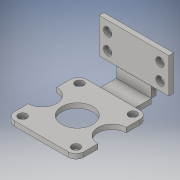
# Autodesk Inventor part: motor mount
Saved by Autodesk Inventor 2016 (Build 200138000, 138)
## iProperties
Created: 2017-09-13
Part Number: motor mount
Material: Generic
Document SubType Name: Modeling
Designer: student
Density: 1 g/cm^3
Appearance: Default
Author: student
Autodesk Inventor part; units mm, degrees
ref_plane "YZ Plane" through (0, 0, 0) normal (1, 0, 0) x (0, 1, 0)
ref_plane "XZ Plane" through (0, 0, 0) normal (0, 1, 0) x (-1, 0, 0)
ref_plane "XY Plane" through (0, 0, 0) normal (0, 0, 1) x (1, 0, 0)
sketch "Sketch1" plane through (0, 0, 0) normal (0, 0, 1) x (1, 0, 0)
  line L0 (-11.0744, 5.588) -> (11.0744, 5.588)
  line L1 (11.0744, 5.588) -> (11.0744, -5.588)
  line L2 (11.0744, -5.588) -> (-11.0744, -5.588)
  line L3 (-11.0744, -5.588) -> (-11.0744, 5.588)
  circle A0 centre (-8.3312, 2.4384) radius 1.3462
  circle A1 centre (8.3312, 2.4384) radius 1.3462
  circle A2 centre (8.3312, -2.794) radius 1.3462
  circle A3 centre (-8.3312, -2.794) radius 1.3462
  point P0 (0, 0)
  dimension "d0" = 22.1488
  dimension "d1" = 11.176
  dimension "d2" = 2.6924
  dimension "d3" = 2.6924
  dimension "d4" = 2.6924
  dimension "d5" = 2.6924
  dimension "d6" = 3.1496
  dimension "d7" = 2.794
  dimension "d8" = 5.2324
  dimension "d9" = 2.7432
  dimension "d10" = 2.7432
  dimension "d11" = 3.1496
  dimension "d12" = 2.794
  constraints: 8 end point, 4 centre point, 2 parallel, 2 vertical alignment, 1 horizontal, 1 perpendicular
  measures "d0" distance of L1.end L2.end
  measures "d1" distance of L1.end L0.end
  measures "d2" diameter of A0
  measures "d3" diameter of A1
  measures "d4" diameter of A2
  measures "d5" diameter of A3
  measures "d6" distance from line of L0 A1.centre
  measures "d7" distance from line of L2 A2.centre
  measures "d8" distance of A2.centre A1.centre
  measures "d9" distance from line of L1 A1.centre
  measures "d10" distance from line of L3 A0.centre
  measures "d11" vertical distance of L0.start A0.centre
  measures "d12" distance from line of L2 A3.centre
extrude "Extrusion1" add sketch "Sketch1" along normal blind 1.524
sketch "Sketch2" plane through (-11.0744, -5.588, 0) normal (0, -1, 0) x (1, 0, 0)
  line L0 (5.5245, 1.5517) -> (16.6243, 1.5517)
  line L1 (16.6243, 1.5517) -> (16.6243, 0.0277)
  line L2 (16.6243, 0.0277) -> (5.5245, 0.0277)
  line L3 (5.5245, 0.0277) -> (5.5245, 1.5517)
  point P0 (11.0744, 0)
  dimension "d15" = 11.0998
  dimension "d16" = 1.524
  constraints: 8 end point, 2 parallel, 1 horizontal, 1 perpendicular
  measures "d15" distance of L1.end L2.end
  measures "d16" distance of L1.end L0.end
extrude "Extrusion2" add sketch "Sketch2" along normal blind 3.3782
sketch "Sketch3" plane through (-5.5499, -5.588, 1.5517) normal (0, 0, 1) x (1, 0, 0)
  line L0 (0, -3.3922) -> (11.0998, -3.3922)
  line L1 (11.0998, -3.3922) -> (11.0998, -4.9162)
  line L2 (11.0998, -4.9162) -> (0, -4.9162)
  line L3 (0, -4.9162) -> (0, -3.3922)
  point P0 (5.5499, 5.588)
  dimension "d19" = 11.0998
  dimension "d20" = 1.524
  constraints: 8 end point, 2 parallel, 1 horizontal, 1 perpendicular
  measures "d19" distance of L1.end L2.end
  measures "d20" distance of L1.end L0.end
extrude "Extrusion3" add sketch "Sketch3" along normal blind 6.4008
sketch "Sketch4" plane through (-5.5499, -8.9802, 1.5517) normal (0, 1, 0) x (1, 0, 0)
  line L0 (14.0462, -29.432) -> (-2.9464, -29.432)
  line L1 (-2.9464, -6.5466) -> (14.0462, -6.5466)
  line L2 (-5.5245, 1.5517) -> (16.6243, 1.5517) projected
  arc A0 (-5.4864, -22.5228) -> (-5.4864, -13.4559) centre (-5.5498, -17.9893) ccw
  arc A1 (16.5862, -13.4558) -> (16.5862, -22.5229) centre (16.6412, -17.9893) ccw
  line L3 (16.5862, -9.0866) -> (16.5862, -13.4558)
  line L4 (16.5862, -22.5229) -> (16.5862, -26.892)
  line L5 (-5.4864, -26.892) -> (-5.4864, -22.5228)
  line L6 (-5.4864, -13.4559) -> (-5.4864, -9.0866)
  circle A2 centre (5.5499, -17.9893) radius 4.9657
  arc A3 (14.0462, -29.432) -> (16.5862, -26.892) centre (14.0462, -26.892) ccw
  arc A4 (-5.4864, -26.892) -> (-2.9464, -29.432) centre (-2.9464, -26.892) ccw
  arc A5 (16.5862, -9.0866) -> (14.0462, -6.5466) centre (14.0462, -9.0866) ccw
  arc A6 (-2.9464, -6.5466) -> (-5.4864, -9.0866) centre (-2.9464, -9.0866) ccw
  circle A7 centre (14.0462, -26.892) radius 1.3208
  circle A8 centre (14.0462, -8.8085) radius 1.3208
  circle A9 centre (-2.9464, -8.8085) radius 1.3208
  circle A10 centre (-2.9464, -26.892) radius 1.3208
  point P0 (5.5499, 1.5517)
  point P1 (-5.4864, -6.5466)
  point P2 (-5.4864, -29.432)
  point P3 (16.5862, -6.5466)
  point P4 (5.5499, 1.5517)
  point P5 (16.5862, -17.9893)
  point P6 (5.5499, 1.5517)
  dimension "d25" = 9.0678
  dimension "d26" = 9.0678
  dimension "d27" = 9.9314
  dimension "d28" = 2.54
  dimension "d29" = 2.6416
  dimension "d30" = 2.6416
  dimension "d31" = 2.6416
  dimension "d32" = 2.6416
  dimension "d33" = 2.54
  constraints: 12 end point, 12 point on circle, 11 centre point, 8 tangent, 6 point on line, 5 parallel, 3 equal radius, 3 horizontal alignment, 3 vertical alignment, 2 coincident, 2 midpoint, 2 perpendicular, 1 horizontal
  measures "d25" diameter of A0
  measures "d26" diameter of A1
  measures "d27" diameter of A2
  measures "d28" radius of A3
  measures "d29" diameter of A7
  measures "d30" diameter of A8
  measures "d31" diameter of A9
  measures "d32" diameter of A10
  measures "d33" distance from line of L0 A4.centre
extrude "Extrusion4" add sketch "Sketch4" along normal blind 1.524
body "Solid1"
